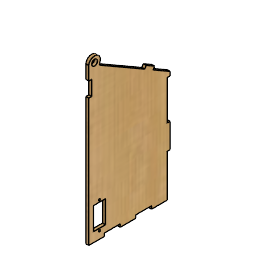
GREENHOUSE ASSEMBLY ALTERED (Autodesk Fusion 360 archive; units mm, degrees)
design "RIght"
Autodesk Fusion 360 part; units mm, degrees
(part 1 of 25)
sketch "Sketch1" plane through (150, 0, 0) normal (1, 0, 0) x (0, 1, 0)
  line L0 (64, 0) -> (80, 0)
  line L1 (80, 0) -> (80, 3)
  line L2 (80, 3) -> (64, 3) construction
  line L3 (0, 3) -> (0, 0)
  line L4 (0, 3) -> (0, 160)
  line L5 (0, 160) -> (83, 112.0799)
  line L6 (80, 3) -> (80, 108.0799)
  line L7 (80, 108.0799) -> (83, 108.0799)
  line L8 (83, 108.0799) -> (83, 112.0799)
  circle A0 centre (5.9574, 158.3503) radius 2.9841
  line L9 (4.524, 160.9676) -> (8.9408, 158.4176) construction
  line L10 (8.9408, 158.4176) -> (7.3908, 155.7329) construction
  line L11 (7.3908, 155.7329) -> (2.974, 158.2829) construction
  line L12 (2.974, 158.2829) -> (4.524, 160.9676) construction
  arc A1 (11.1398, 155.3582) -> (0, 157.7854) centre (5.9574, 158.3503) ccw
  line L13 (-5.009, 151.3242) -> (0, 160) construction
  line L14 (11.1398, 155.3582) -> (10.3648, 154.0159) construction
  arc A2 (11.1398, 155.3582) -> (11.7071, 153.2409) centre (12.4821, 154.5832) ccw
  line L15 (64, 3) -> (64, 0)
  line L16 (0, 0) -> (16, 0)
  line L17 (16, 0) -> (16, 3)
  line L18 (80, 0) -> (80, 3)
  line L19 (64, 0) -> (80, 0)
  line L20 (64, 0) -> (64, 3)
  line L21 (48, 3) -> (64, 3)
  line L22 (48, 0) -> (48, 3)
  line L23 (32, 0) -> (48, 0)
  line L24 (32, 0) -> (32, 3)
  line L25 (16, 3) -> (32, 3)
  line L26 (57.0192, 127.0799) -> (58.5192, 129.678)
  line L27 (58.5192, 129.678) -> (67.1795, 124.678)
  line L28 (67.1795, 124.678) -> (65.6795, 122.0799)
  line L29 (0, 145) -> (3, 145)
  line L30 (3, 145) -> (3, 130)
  line L31 (3, 130) -> (0, 130)
  line L32 (80, 68.04) -> (83, 68.04)
  line L33 (83, 68.04) -> (83, 43.04)
  line L34 (83, 43.04) -> (80, 43.04)
  line L35 (83, 55.54) -> (80, 55.54) construction
  dimension "d13" = 60
  dimension "d14" = 160
  dimension "d22" = 3
  dimension "d23" = 4
  dimension "d24" = 3.1
  dimension "d25" = 5.1
  dimension "d26" = 3
  dimension "d45" = 3
  dimension "d46" = 10
  dimension "d47" = 20
  dimension "d54" = 3
  dimension "d55" = 15
  dimension "d56" = 15
  dimension "d60" = 25
  constraint perpendicular L2 L4
  constraint coincident L1.end L2.start
  constraint perpendicular L2 L6
  constraint perpendicular L6 L7
  constraint perpendicular L7 L8
  constraint perpendicular L9 L10
  constraint parallel L9 L11
  constraint parallel L10 L12
  constraint coincident A0 L9.end
  constraint coincident A0 L9.start
  constraint coincident A0 L10.end
  constraint collinear L5 L11
  constraint coincident A0.centre A1.centre
  constraint coincident L5 L14.end
  constraint tangent A1 L14
  constraint perpendicular L5 L13
  constraint perpendicular L5 L14
  constraint tangent A1 L13
  constraint coincident L4 A1.end
  constraint tangent A1 A2
  constraint tangent L5 A2
  constraint coincident L5 A2.end
  constraint coincident L3.start L4.start
  constraint coincident L5 L26.start
  constraint perpendicular L5 L26
  constraint perpendicular L26 L27
  constraint coincident L5 L28.end
  constraint perpendicular L5 L28
  constraint coincident L4 L29.start
  constraint perpendicular L4 L29
  constraint perpendicular L29 L30
  constraint coincident L4 L31.end
  constraint perpendicular L4 L31
  constraint coincident L6 L32.start
  constraint perpendicular L6 L32
  constraint perpendicular L32 L33
  constraint coincident L6 L34.end
  constraint perpendicular L6 L34
  constraint collinear L8 L33
  constraint midpoint L33 L35.start
  constraint midpoint L6 L35.end
  constraint perpendicular L33 L35
  measures "d13" angle of L4 L5
  measures "d14" distance of L3.end L4.end
  measures "d22" distance of L6.end L7.end
  measures "d23" distance of L5.end L7.end
  measures "d24" distance of L9.end L10.end
  measures "d25" distance of L9.start L9.end
  measures "d26" distance of A0 A1
  measures "d45" distance of L26.start L26.end
  measures "d46" distance of L26.end L27.end
  measures "d47" distance of L5.end L28
  measures "d54" distance of L29.start L29.end
  measures "d55" distance of L29.end L30.end
  measures "d56" distance of L4.end L29
  measures "d60" distance of L32.end L33.end
extrude "Extrude1" add sketch "Sketch1" along normal blind 3 contours L0 L1 L3 L4 L5 L6 L7 L8 A0 A1 L15 L16 L17 L18 L19 L20 L21 L22 L23 L24 L25 L29 L30 L31 | L6 L32 L33 L34 | L5 L26 L27 L28 | L5 A0 A1 A2
sketch "Sketch2" plane through (153, 0, 0) normal (1, 0, 0) x (0, 1, 0)
  circle A0 centre (5.9574, 158.3503) radius 2.9841
  line L0 (80, 68.04) -> (80, 108.0799)
  line L1 (80, 108.0799) -> (83, 108.0799)
  line L2 (83, 108.0799) -> (83, 112.0799)
  line L3 (83, 112.0799) -> (65.6795, 122.0799)
  line L4 (65.6795, 122.0799) -> (67.1795, 124.678)
  line L5 (67.1795, 124.678) -> (58.5192, 129.678)
  line L6 (58.5192, 129.678) -> (57.0192, 127.0799)
  line L7 (57.0192, 127.0799) -> (11.7071, 153.2409)
  arc A1 (11.1398, 155.3582) -> (11.7071, 153.2409) centre (12.4821, 154.5832) ccw
  arc A2 (11.1398, 155.3582) -> (0, 158.9152) centre (5.9574, 158.3503) ccw
  line L8 (0, 158.9152) -> (0, 145)
  line L9 (0, 145) -> (3, 145)
  line L10 (3, 145) -> (3, 130)
  line L11 (3, 130) -> (0, 130)
  line L12 (0, 130) -> (0, 0)
  line L13 (0, 0) -> (16, 0)
  line L14 (16, 0) -> (16, 3)
  line L15 (16, 3) -> (32, 3)
  line L16 (32, 3) -> (32, 0)
  line L17 (32, 0) -> (48, 0)
  line L18 (48, 0) -> (48, 3)
  line L19 (48, 3) -> (64, 3)
  line L20 (64, 3) -> (64, 0)
  line L21 (64, 0) -> (80, 0)
  line L22 (80, 0) -> (80, 43.04)
  line L23 (80, 43.04) -> (83, 43.04)
  line L24 (83, 43.04) -> (83, 68.04)
  line L25 (83, 68.04) -> (80, 68.04)
  arc A3 (10.3278, 35.6711) -> (11.6278, 35.6711) centre (10.9778, 34.9111) ccw
  arc A4 (11.6278, 6.8512) -> (10.3278, 6.8512) centre (10.9778, 7.6111) ccw
  arc A5 (10.3278, 6.8512) -> (11.6278, 6.8512) centre (10.9778, 7.6111) ccw
  arc A6 (11.6278, 35.6711) -> (10.3278, 35.6711) centre (10.9778, 34.9111) ccw
  line L26 (16.8528, 26.6361) -> (16.8528, 10.0111) construction
  line L27 (16.8528, 32.5111) -> (16.8528, 26.6361) construction
  line L28 (10.9778, 32.5111) -> (16.8528, 32.5111) construction
  line L29 (5.1028, 32.5111) -> (10.9778, 32.5111) construction
  line L30 (5.1028, 26.6361) -> (5.1028, 32.5111) construction
  line L31 (5.1028, 10.0111) -> (5.1028, 26.6361) construction
  line L32 (5.1028, 10.0111) -> (16.8528, 10.0111) construction
  line L33 (4.9028, 9.8111) -> (17.0528, 9.8111)
  line L34 (17.0528, 26.6361) -> (17.0528, 9.8111)
  line L35 (17.0528, 32.7111) -> (17.0528, 26.6361)
  line L36 (10.9778, 32.7111) -> (17.0528, 32.7111)
  line L37 (4.9028, 32.7111) -> (10.9778, 32.7111)
  line L38 (4.9028, 26.6361) -> (4.9028, 32.7111)
  line L39 (4.9028, 9.8111) -> (4.9028, 26.6361)
  dimension "d94" = 0.2
  constraint coincident A4.start A5.end
  constraint coincident A4.centre A5.centre
  constraint coincident A3.end A6.start
  constraint coincident A3.centre A6.centre
  constraint coincident A3.start A6.end
  constraint coincident A4.end A5.start
extrude "Extrude2" cut sketch "Sketch2" against normal up to surface (3 mm away) contours A3 A6 | A4 A5 | L33 L34 L35 L36 L37 L38 L39

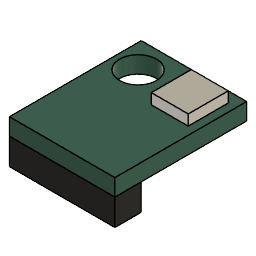
design "BMP180"
Autodesk Fusion 360 part; units mm, degrees
sketch "Sketch1" plane through (0, 0, 0) normal (0, 0, 1) x (1, 0, 0)
  line L0 (0, 0) -> (10, 0)
  line L1 (10, 0) -> (10, 12.5)
  line L2 (10, 12.5) -> (0, 12.5)
  line L3 (0, 12.5) -> (0, 0)
  circle A0 centre (2.25, 9.95) radius 1.75
  line L4 (5.75, 11.5) -> (9.25, 11.5)
  line L5 (9.25, 11.5) -> (9.25, 7.7)
  line L6 (9.25, 7.7) -> (5.75, 7.7)
  line L7 (5.75, 7.7) -> (5.75, 11.5)
  line L8 (10, 2.5) -> (0, 2.5)
  dimension "d1" = 10
  dimension "d2" = 12.5
  dimension "d3" = 3.5
  dimension "d4" = 2.55
  dimension "d5" = 2.25
  dimension "d6" = 3.5
  dimension "d7" = 3.8
  dimension "d8" = 0.75
  dimension "d9" = 1
  dimension "d10" = 2.5
  constraint horizontal L0
  constraint vertical L1
  constraint horizontal L2
  constraint vertical L3
  constraint coincident L0.start L3.end
  constraint horizontal L4
  constraint vertical L5
  constraint horizontal L6
  constraint vertical L7
  constraint coincident L1 L8.start
  constraint coincident L3 L8.end
  constraint perpendicular L3 L8
  measures "d1" distance of L0.start L0.end
  measures "d2" distance of L0.start L2.end
  measures "d3" diameter of A0
  measures "d4" distance of L2 A0.centre
  measures "d5" distance of L3 A0.centre
  measures "d6" distance of L4.start L4.end
  measures "d7" distance of L4.start L6.end
  measures "d8" distance of L1 L5
  measures "d9" distance of L2 L4
  measures "d10" distance of L0 L8
extrude "Extrude1" add sketch "Sketch1" along normal blind 1.6 contours L0 L1 L3 L8 | L1 L2 L3 L8 | L4 L5 L6 L7 makes body 1
extrude "Extrude2" add sketch "Sketch1" along normal blind 1 from surface at 1.6 separate body contours L4 L5 L6 L7 makes body 2
extrude "Extrude3" add sketch "Sketch1" against normal blind 2.5 separate body contours L0 L1 L3 L8 makes body 3
equation "d4 = d3 / 2 + 0.8 mm"
equation "d5 = d3 / 2 + 0.5 mm"

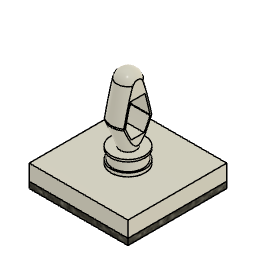
design "PCB Support Pin"
Autodesk Fusion 360 part; units mm, degrees
sketch "Sketch1" plane through (0, 0, 0) normal (0, 0, 1) x (1, 0, 0)
  line L0 (6.35, 6.35) -> (-6.35, 6.35)
  line L1 (-6.35, 6.35) -> (-6.35, -6.35)
  line L2 (-6.35, -6.35) -> (6.35, -6.35)
  line L3 (6.35, -6.35) -> (6.35, 6.35)
  line L4 (6.35, 6.35) -> (-6.35, -6.35) construction
  line L5 (-6.35, 6.35) -> (6.35, -6.35) construction
  dimension "d1" = 12.7
  dimension "d2" = 12.7
  constraint horizontal L0
  constraint perpendicular L0 L1
  constraint parallel L0 L2
  constraint parallel L1 L3
  constraint coincident L4 origin
  constraint coincident L5 origin
  measures "d1" distance of L1.end L2.end
  measures "d2" distance of L0.end L1.end
extrude "Extrude1" add sketch "Sketch1" along normal blind 2.032 makes body 1
extrude "Extrude2" add 1 faces at (-2.1167, -2.1167, 0) along direction (0, 0, -1) blind 0.8 separate body on bodies 1 makes body 2
sketch "Sketch2" plane through (0, 0, 0) normal (0, 1, 0) x (1, 0, 0)
  line L0 (-6.35, -2.032) -> (6.35, -2.032)
  line L1 (0, -2.032) -> (0, -12.6938)
  line L2 (0, -3.9625) -> (2.1828, -3.9625)
  line L3 (2.1828, -3.9625) -> (2.1828, -3.6971)
  line L4 (2.1828, -3.6971) -> (1.9857, -3.6971)
  line L5 (1.9857, -3.6971) -> (1.9857, -2.4654)
  line L6 (1.9857, -2.4654) -> (2.1828, -2.4654)
  line L7 (2.1828, -2.4654) -> (2.1828, -2.032)
  line L8 (6.35, 0.8) -> (-6.35, 0.8) construction
  line L9 (1.0176, -3.9625) -> (2.1587, -7.0975)
  line L10 (2.1763, -7.3064) -> (1.4028, -11.5248)
  arc A0 (0, -12.6938) -> (1.4028, -11.5248) centre (0, -11.2676) ccw
  arc A1 (2.1763, -7.3064) -> (2.1587, -7.0975) centre (1.7828, -7.2343) ccw
  line L11 (0, -12.6938) -> (1.1885, -12.6938) construction
  line L12 (1.1885, -12.6938) -> (1.4028, -11.5248) construction
  line L13 (2.1828, -3.9625) -> (2.1828, -7.2343) construction
  line L14 (1.6, -3.9625) -> (1.6, -5.5625) construction
  line L15 (1.6, -5.5625) -> (0, -5.5625) construction
  arc A2 (1.9795, -7.2704) -> (1.9708, -7.1659) centre (1.7828, -7.2343) ccw
  line L16 (0.8297, -4.0309) -> (0.8048, -3.9625)
  dimension "d7" = 4.7625
  dimension "d8" = 4.3656
  dimension "d10" = 0.4
  dimension "d11" = 8.7313
  dimension "d12" = 3.2
  dimension "d13" = 1.6
  dimension "d15" = 70
  constraint midpoint L0 L1.start
  constraint perpendicular L0 L1
  constraint perpendicular L1 L2
  constraint perpendicular L2 L3
  constraint perpendicular L3 L4
  constraint perpendicular L4 L5
  constraint perpendicular L5 L6
  constraint coincident L0 L7.end
  constraint perpendicular L0 L7
  constraint collinear L3 L7
  constraint coincident L2.start L1
  constraint coincident L1.end A0.start
  constraint tangent L10 A0
  constraint tangent L9 A1
  constraint tangent L10 A1
  constraint perpendicular L1 L11
  constraint tangent A0 L12
  constraint tangent A0 L11
  constraint coincident A1 L13.end
  constraint tangent A1 L13
  constraint perpendicular L2 L13
  constraint coincident L2 L9.start
  constraint coincident L2 L14.start
  constraint coincident L9 L14.end
  constraint perpendicular L2 L14
  constraint coincident L1 L15.end
  constraint perpendicular L1 L15
  constraint coincident L2 L16.end
  constraint concentric A1 A2
  measures "d7" distance of L2 L8
  measures "d10" radius of A1
  measures "d11" distance of L2 L1.end
  measures "d13" distance of L14.start L14.end
  measures "d15" angle of L2 L9
revolve "Revolve1" add sketch "Sketch2" angle 360 about axis through (0, 0, 2.032) along (0, 0, 1) bodies 1
sketch "Sketch3" plane through (0, 0, 0) normal (0, 1, 0) x (1, 0, 0)
  line L0 (-2.1828, -3.9625) -> (2.1828, -3.9625)
  arc A0 (-1.4028, -11.5248) -> (0, -12.6938) centre (0, -11.2676) ccw
  arc A1 (0, -12.6938) -> (1.4028, -11.5248) centre (0, -11.2676) ccw
  line L1 (1.25, -3.9625) -> (1.25, -12.6938)
  line L2 (1.25, -12.6938) -> (-1.25, -12.6938)
  line L3 (-1.25, -12.6938) -> (-1.25, -3.9625)
  line L4 (2.1828, -3.9625) -> (2.1828, -12.6938)
  line L5 (2.1828, -12.6938) -> (1.25, -12.6938)
  line L6 (-1.25, -12.6938) -> (-2.1828, -12.6938)
  line L7 (-2.1828, -12.6938) -> (-2.1828, -3.9625)
  dimension "d16" = 2.5
  constraint coincident L0 L1.start
  constraint perpendicular L0 L1
  constraint perpendicular L1 L2
  constraint coincident L0 L3.end
  constraint perpendicular L0 L3
  constraint midpoint A0.end L2
  constraint coincident L0.end L4.start
  constraint perpendicular L0 L4
  constraint perpendicular L1 L5
  constraint perpendicular L3 L6
  constraint coincident L0.start L7.end
  constraint perpendicular L0 L7
  measures "d16" distance of L1.end L2.end
extrude "Extrude3" cut sketch "Sketch3" along normal through all and the other way through all contours L0 L3 L6 L7 | L0 L1 L4 L5 bodies 1
sketch "Sketch4" plane through (1.25, 0, 0) normal (1, 0, 0) x (0, 1, 0)
  arc A0 (0.6367, 11.5248) -> (-0.6367, 11.5248) centre (0, 11.2676) ccw
  spline S0 degree 2 poles (-1.7815, 7.3064) (-1.0854, 10.4141) (-0.6367, 11.5248) knots 0 0 0 0.437351 0.437351 0.437351 weights 1 1.055449 1
  spline S1 degree 3 poles (-1.76, 7.0975) (-1.7782, 7.1383) (-1.7895, 7.19) (-1.7895, 7.2343) (-1.7895, 7.2572) (-1.7869, 7.2821) (-1.7815, 7.3064) knots -0.013287 -0.013287 -0.013287 -0.013287 0 0 0 0.006866 0.006866 0.006866 0.006866
  spline S2 degree 2 poles (0, 4.6009) (-0.6454, 4.6009) (-1.76, 7.0975) knots 0.311685 0.311685 0.311685 0.623369 0.623369 0.623369 weights 1 1.16768 1
  spline S3 degree 2 poles (1.76, 7.0975) (0.6454, 4.6009) (0, 4.6009) knots 0 0 0 0.311685 0.311685 0.311685 weights 1 1.16768 1
  spline S4 degree 3 poles (1.7815, 7.3064) (1.7869, 7.2821) (1.7895, 7.2572) (1.7895, 7.2343) (1.7895, 7.19) (1.7782, 7.1383) (1.76, 7.0975) knots -0.006866 -0.006866 -0.006866 -0.006866 0 0 0 0.013287 0.013287 0.013287 0.013287
  spline S5 degree 2 poles (0.6367, 11.5248) (1.0854, 10.4141) (1.7815, 7.3064) knots 0 0 0 0.437351 0.437351 0.437351 weights 1 1.055449 1
  spline S6 degree 3 poles (1.5773, 7.179) (1.0909, 6.0894) (0.7682, 5.5108) (0.4944, 5.1632) (0.2828, 4.8944) (0.1228, 4.8009) (0, 4.8009) knots 0 0 0 0 0.17577 0.17577 0.17577 0.311685 0.311685 0.311685 0.311685
  spline S7 degree 3 poles (0, 4.8009) (-0.1696, 4.8009) (-0.4174, 4.9925) (-0.7546, 5.5437) (-0.9772, 5.9076) (-1.2343, 6.4106) (-1.5773, 7.179) knots 0.311685 0.311685 0.311685 0.311685 0.499423 0.499423 0.499423 0.623369 0.623369 0.623369 0.623369
  spline S8 degree 3 poles (-1.5773, 7.179) (-1.5825, 7.1906) (-1.5895, 7.2239) (-1.5895, 7.2343) (-1.5895, 7.2423) (-1.5883, 7.2538) (-1.5863, 7.2627) knots -0.013287 -0.013287 -0.013287 -0.013287 0 0 0 0.006866 0.006866 0.006866 0.006866
  spline S9 degree 3 poles (-1.5863, 7.2627) (-1.1749, 9.0993) (-0.8714, 10.2577) (-0.6005, 11.0468) (-0.5494, 11.1956) (-0.4997, 11.3299) (-0.4512, 11.4499) knots 0 0 0 0 0.367958 0.367958 0.367958 0.437351 0.437351 0.437351 0.437351
  arc A1 (0.4512, 11.4499) -> (-0.4512, 11.4499) centre (0, 11.2676) ccw
  spline S10 degree 3 poles (0.4512, 11.4499) (0.7082, 10.8137) (0.9931, 9.8115) (1.3651, 8.2283) (1.4352, 7.9297) (1.5087, 7.6091) (1.5863, 7.2627) knots 0 0 0 0 0.367958 0.367958 0.367958 0.437351 0.437351 0.437351 0.437351
  spline S11 degree 3 poles (1.5863, 7.2627) (1.5883, 7.2538) (1.5895, 7.2423) (1.5895, 7.2343) (1.5895, 7.2239) (1.5825, 7.1906) (1.5773, 7.179) knots -0.006866 -0.006866 -0.006866 -0.006866 0 0 0 0.013287 0.013287 0.013287 0.013287
  line L0 (0.8161, 5.6442) -> (-0.8149, 5.6442)
  line L1 (0.9353, 9.9416) -> (-0.9355, 9.9416)
  dimension "d18" = 0.2
  constraint coincident S6 L0.start
  constraint coincident S7 L0.end
  constraint horizontal L0
  constraint coincident S10 L1.start
  constraint coincident S9 L1.end
  constraint parallel L0 L1
extrude "Extrude4" cut sketch "Sketch4" against normal through all contours S6 S7 S8 S9 S10 S11 L0 L1 bodies 1
equation "d7 = 3\" / 16"
equation "d8 = 11\" / 64"
equation "d11 = 11\" / 32"

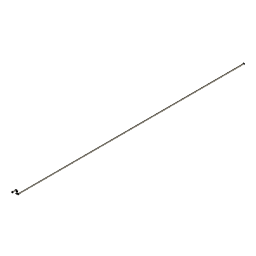
design "Push Rod"
Autodesk Fusion 360 part; units mm, degrees
sketch "Sketch1" plane through (0, 0, 0) normal (1, 0, 0) x (0, 1, 0)
  line L0 (0, 0) -> (3, 0)
  line L1 (4, -1) -> (4, -3)
  line L2 (5, -4) -> (204, -4)
  arc A0 (4, -1) -> (3, 0) centre (3, -1) ccw
  arc A1 (4, -3) -> (5, -4) centre (5, -3) ccw
  point P0 (4, 0)
  point P1 (4, -4)
  dimension "d1" = 4
  dimension "d2" = 4
  dimension "d3" = 200
  dimension "d4" = 1
  dimension "d5" = 1
  constraint coincident L0.start origin
  constraint horizontal L0
  constraint perpendicular L0 L1
  constraint perpendicular L1 L2
  constraint coincident P0 L0
  constraint coincident P0 L1
  constraint tangent L0 A0
  constraint tangent L1 A0
  constraint coincident P1 L1
  constraint coincident P1 L2
  constraint tangent L1 A1
  constraint tangent L2 A1
  measures "d1" distance of L0.start P0
  measures "d2" distance of P0 P1
  measures "d3" distance of P1 L2.end
  measures "d4" radius of A0
  measures "d5" radius of A1
sketch "Sketch2" plane through (0, 0, 0) normal (0, 1, 0) x (1, 0, 0)
  circle A0 centre (0, 0) radius 0.6
  dimension "d6" = 1.2
  constraint coincident A0.centre origin
  measures "d6" diameter of A0
sweep "Sweep1" add profiles "Sketch2" path "Sketch1" along L0 A0 L1 A1 L2 section 1

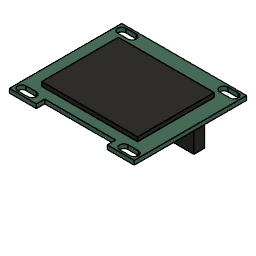
design "oled"
description: IIC OLED 0.96" 4Pin SSD1306
part number: GME12864-11
Autodesk Fusion 360 part; units mm, degrees
sketch "Sketch1" plane through (0, 0, 0) normal (0, 1, 0) x (1, 0, 0)
  line L0 (0, 0) -> (30, 0)
  line L1 (30, 0) -> (30, -27)
  line L2 (30, -27) -> (0, -27)
  line L3 (0, -27) -> (0, 0)
  line L4 (6.5, -27) -> (6.5, -25)
  line L5 (6.5, -25) -> (23.5, -25)
  line L6 (23.5, -25) -> (23.5, -27)
  line L7 (15, -27) -> (15, -25) construction
  line L8 (3.5, -4.3) -> (26.5, -4.3)
  line L9 (26.5, -4.3) -> (26.5, -22.7)
  line L10 (26.5, -22.7) -> (3.5, -22.7)
  line L11 (3.5, -22.7) -> (3.5, -4.3)
  line L12 (1.5, -2.5) -> (4, -2.5)
  arc A0 (4, -2.5) -> (4, -0.5) centre (4, -1.5) ccw
  line L13 (4, -0.5) -> (1.5, -0.5)
  arc A1 (1.5, -0.5) -> (1.5, -2.5) centre (1.5, -1.5) ccw
  line L14 (1.5, -1.5) -> (4, -1.5) construction
  line L15 (15, 0) -> (15, -25) construction
  line L16 (0, -13.5) -> (30, -13.5) construction
  arc A2 (26, -0.5) -> (26, -2.5) centre (26, -1.5) ccw
  line L17 (26, -0.5) -> (28.5, -0.5)
  arc A3 (28.5, -2.5) -> (28.5, -0.5) centre (28.5, -1.5) ccw
  line L18 (28.5, -2.5) -> (26, -2.5)
  line L19 (26, -26.5) -> (28.5, -26.5)
  arc A4 (28.5, -26.5) -> (28.5, -24.5) centre (28.5, -25.5) ccw
  line L20 (28.5, -24.5) -> (26, -24.5)
  arc A5 (26, -24.5) -> (26, -26.5) centre (26, -25.5) ccw
  line L21 (4, -26.5) -> (1.5, -26.5)
  arc A6 (4, -26.5) -> (4, -24.5) centre (4, -25.5) ccw
  arc A7 (1.5, -24.5) -> (1.5, -26.5) centre (1.5, -25.5) ccw
  line L22 (1.5, -24.5) -> (4, -24.5)
  dimension "d1" = 30
  dimension "d2" = 27
  dimension "d3" = 6.5
  dimension "d4" = 2
  dimension "d5" = 3.5
  dimension "d6" = 3.5
  dimension "d7" = 4.3
  dimension "d8" = 4.3
  dimension "d22" = 1.5
  dimension "d23" = 1.5
  dimension "d24" = 1
  dimension "d25" = 2.5
  constraint horizontal L0
  constraint vertical L1
  constraint horizontal L2
  constraint vertical L3
  constraint coincident L0.start L3.end
  constraint coincident L2 L4.start
  constraint perpendicular L2 L4
  constraint perpendicular L4 L5
  constraint coincident L2 L6.end
  constraint perpendicular L2 L6
  constraint midpoint L2 L7.start
  constraint midpoint L5 L7.end
  constraint perpendicular L2 L7
  constraint horizontal L8
  constraint vertical L9
  constraint horizontal L10
  constraint vertical L11
  constraint tangent L12 A0
  constraint tangent A0 L13
  constraint parallel L12 L13
  constraint tangent L13 A1
  constraint tangent L12 A1
  constraint horizontal L14
  constraint midpoint L0 L15.start
  constraint midpoint L3 L16.start
  constraint midpoint L1 L16.end
  constraint symmetric L12.start L15 A3.start
  constraint symmetric L12.end L15 A2.end
  constraint symmetric A0.end L15 A2.start
  constraint symmetric L13.end L15 L17.end
  constraint symmetric A0 L15 A2
  constraint symmetric A1 L15 A3
  constraint symmetric L12.start L16 A7.start
  constraint symmetric L12.end L16 A6.end
  constraint symmetric A0.end L16 L21.start
  constraint symmetric L13.end L16 L21.end
  constraint symmetric A0 L16 A6
  constraint symmetric A1 L16 A7
  constraint symmetric L16 A2.end L20.end
  constraint symmetric L16 A2.start L19.start
  constraint symmetric L16 A2 A5
  constraint symmetric L16 L17.end L19.end
  constraint symmetric L16 A3.start A4.end
  constraint symmetric L16 A3 A4
  measures "d1" distance of L0.start L0.end
  measures "d2" distance of L0.start L2.end
  measures "d3" distance of L1 L6
  measures "d4" distance of L2 L5
  measures "d5" distance of L1 L9
  measures "d6" distance of L3 L11
  measures "d7" distance of L0 L8
  measures "d8" distance of L2 L10
  measures "d22" distance of L3 A1.centre
  measures "d23" distance of L0 A1.centre
  measures "d24" radius of A1
  measures "d25" distance of A1.centre A0.centre
extrude "Extrude1" add sketch "Sketch1" along normal blind 1 contours L8 L9 L10 L11 makes body 1
extrude "Extrude2" add sketch "Sketch1" against normal blind 1 separate body contours L0 L1 L2 L3 L4 L5 L6 | L8 L9 L10 L11 makes body 2
sketch "Sketch2" plane through (0, -1, 0) normal (0, -1, 0) x (1, 0, 0)
  line L0 (6.5, 25) -> (6.5, 27)
  line L1 (6.5, 27) -> (0, 27)
  line L2 (0, 27) -> (0, 0)
  line L3 (0, 0) -> (30, 0)
  line L4 (30, 0) -> (30, 27)
  line L5 (30, 27) -> (23.5, 27)
  line L6 (23.5, 27) -> (23.5, 25)
  line L7 (23.5, 25) -> (6.5, 25)
  line L8 (10.1, 2.6) -> (19.9, 2.6)
  line L9 (19.9, 2.6) -> (19.9, 0)
  line L10 (10.1, 0) -> (10.1, 2.6)
  line L11 (15, 0) -> (15, 2.6) construction
  arc A0 (26, 2.5) -> (26, 0.5) centre (26, 1.5) ccw
  line L12 (26, 2.5) -> (28.5, 2.5)
  arc A1 (28.5, 0.5) -> (28.5, 2.5) centre (28.5, 1.5) ccw
  line L13 (28.5, 0.5) -> (26, 0.5)
  arc A2 (26, 26.5) -> (26, 24.5) centre (26, 25.5) ccw
  line L14 (26, 26.5) -> (28.5, 26.5)
  arc A3 (28.5, 24.5) -> (28.5, 26.5) centre (28.5, 25.5) ccw
  line L15 (28.5, 24.5) -> (26, 24.5)
  arc A4 (4, 24.5) -> (4, 26.5) centre (4, 25.5) ccw
  line L16 (4, 24.5) -> (1.5, 24.5)
  arc A5 (1.5, 26.5) -> (1.5, 24.5) centre (1.5, 25.5) ccw
  line L17 (1.5, 26.5) -> (4, 26.5)
  arc A6 (1.5, 2.5) -> (1.5, 0.5) centre (1.5, 1.5) ccw
  line L18 (1.5, 2.5) -> (4, 2.5)
  arc A7 (4, 0.5) -> (4, 2.5) centre (4, 1.5) ccw
  line L19 (4, 0.5) -> (1.5, 0.5)
  dimension "d13" = 9.8
  dimension "d14" = 2.6
  constraint horizontal L8
  constraint vertical L9
  constraint vertical L10
  constraint midpoint L3 L11.start
  constraint perpendicular L3 L11
  constraint coincident L3 L9.end
  constraint coincident L3 L10.start
  constraint midpoint L8 L11.end
  measures "d13" distance of L8.start L8.end
  measures "d14" distance of L8.start L10.start
extrude "Extrude3" add sketch "Sketch2" along normal blind 15 separate body contours L3 L8 L9 L10 makes body 3
sketch "Minimal Projection" plane through (0, -1, 0) normal (0, -1, 0) x (1, 0, 0)
  arc A0 (26, 2.5) -> (26, 0.5) centre (26, 1.5) ccw
  line L0 (26, 2.5) -> (28.5, 2.5)
  arc A1 (28.5, 0.5) -> (28.5, 2.5) centre (28.5, 1.5) ccw
  line L1 (28.5, 0.5) -> (26, 0.5)
  arc A2 (26, 26.5) -> (26, 24.5) centre (26, 25.5) ccw
  line L2 (26, 26.5) -> (28.5, 26.5)
  arc A3 (28.5, 24.5) -> (28.5, 26.5) centre (28.5, 25.5) ccw
  line L3 (28.5, 24.5) -> (26, 24.5)
  arc A4 (4, 24.5) -> (4, 26.5) centre (4, 25.5) ccw
  line L4 (4, 24.5) -> (1.5, 24.5)
  arc A5 (1.5, 26.5) -> (1.5, 24.5) centre (1.5, 25.5) ccw
  line L5 (1.5, 26.5) -> (4, 26.5)
  arc A6 (1.5, 2.5) -> (1.5, 0.5) centre (1.5, 1.5) ccw
  line L6 (1.5, 2.5) -> (4, 2.5)
  arc A7 (4, 0.5) -> (4, 2.5) centre (4, 1.5) ccw
  line L7 (4, 0.5) -> (1.5, 0.5)
  line L8 (6.5, 25) -> (6.5, 27)
  line L9 (6.5, 27) -> (0, 27)
  line L10 (0, 27) -> (0, 0)
  line L11 (0, 0) -> (30, 0)
  line L12 (30, 0) -> (30, 27)
  line L13 (30, 27) -> (23.5, 27)
  line L14 (23.5, 27) -> (23.5, 25)
  line L15 (23.5, 25) -> (6.5, 25)
  line L16 (19.9, 0) -> (19.9, 2.6)
  line L17 (19.9, 2.6) -> (10.1, 2.6)
  line L18 (10.1, 2.6) -> (10.1, 0)

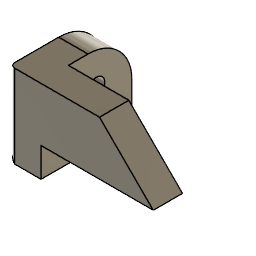
design "MOUNT REAl"
part number: 2026-05-05-22-33-46-720
Autodesk Fusion 360 part; units mm, degrees
sketch "Sketch1" plane through (0, 0, 0) normal (0, 0, 1) x (1, 0, 0)
  line L0 (0, 0) -> (14.68, 0)
  line L1 (14.68, 0) -> (14.68, 3)
  line L2 (14.68, 3) -> (11.68, 3)
  line L3 (11.68, 3) -> (3, 3)
  line L4 (3, 3) -> (3, 9.502)
  line L5 (0, 0) -> (0, 9.502)
  line L6 (0, 9.502) -> (3, 9.502)
  dimension "d4" = 3
  dimension "d5" = 3
  dimension "d6" = 8.68
  dimension "d7" = 6.502
  dimension "d88" = 3
  constraint coincident L0.start L5.start
  constraint horizontal L0
  constraint perpendicular L0 L1
  constraint perpendicular L1 L2
  constraint parallel L2 L3
  constraint perpendicular L3 L4
  constraint perpendicular L0 L5
  constraint perpendicular L4 L6
  measures "d4" distance of L0.end L1.end
  measures "d5" distance of L1.end L2.end
  measures "d6" distance of L2.end L3.end
  measures "d7" distance of L3.end L4.end
  measures "d88" distance of L4.end L5.end
extrude "Extrude18" add sketch "Sketch1" along normal blind 8.5 makes body 1
sketch "Sketch18" plane through (0, 0, 0) normal (0, -1, 0) x (1, 0, 0)
  line L0 (0, 0) -> (14.68, 0)
  line L1 (14.68, 0) -> (14.68, 8.5)
  line L2 (14.68, 8.5) -> (0, 8.5)
  line L3 (0, 8.5) -> (0, 0)
  line L4 (3.2, 0) -> (10.41, 0)
  line L5 (10.41, 0) -> (10.41, 3)
  line L6 (10.41, 3) -> (3.2, 3)
  line L7 (3.2, 3) -> (3.2, 0)
  dimension "d93" = 7.21
  dimension "d94" = 3
  dimension "d95" = 10.41
  constraint perpendicular L4 L5
  constraint perpendicular L5 L6
  constraint perpendicular L4 L7
  constraint coincident L0 L4.start
  constraint coincident L0 L4.end
  measures "d93" distance of L5.end L6.end
  measures "d94" distance of L4.end L5.end
  measures "d95" distance of L3 L5
extrude "Extrude19" cut sketch "Sketch18" against normal blind 3 contours L0 L4 L5 L6 L7 bodies 1
sketch "Sketch19" plane through (0, 0, 0) normal (0, 0, 1) x (1, 0, 0)
  line L0 (1.73, 2) -> (1.73, 8.5)
  line L1 (1.73, 8.5) -> (7.43, 8.5)
  line L2 (7.43, 8.5) -> (7.43, 2)
  line L3 (7.43, 2) -> (1.73, 2)
  dimension "d99" = 5.7
  constraint perpendicular L0 L1
  constraint perpendicular L1 L2
  measures "d99" distance of L0.end L1.end
sketch "Sketch23" plane through (0, 0, 0) normal (-1, 0, 0) x (0, -1, 0)
  line L0 (-9.502, 0) -> (0, 0)
  line L1 (0, 0) -> (0, 8.5)
  line L2 (0, 8.5) -> (-9.502, 8.5)
  line L3 (-9.502, 8.5) -> (-9.502, 0)
  circle A0 centre (-5.852, 5.15) radius 0.8695
  dimension "d107" = 1.739
  dimension "d108" = 3.35
  dimension "d109" = 3.65
  measures "d107" diameter of A0
  measures "d108" distance of L2 A0.centre
  measures "d109" distance of L3 A0.centre
extrude "Extrude23" cut sketch "Sketch23" against normal blind 6.5 contours A0 bodies 1
fillet "Fillet3" radius 4.5 1 edges at (1.5, 9.502, 8.5) on bodies 1
chamfer "Chamfer3" distance 0.5 angle 45 1 edges at (0, 4.751, 0) on bodies 1
fillet "Fillet4" radius 0.5 1 edges at (0, 0, 4.5) on bodies 1
chamfer "Chamfer4" distance 5.5 angle 45 1 edges at (14.68, 1.5, 8.5) on bodies 1
sketch "Sketch24" plane through (0, 0, 0) normal (0, 0, 1) x (1, 0, 0)
  line L0 (3, 3) -> (7, 3)
  line L1 (7, 3) -> (7, 9.5)
  line L2 (7, 9.5) -> (3, 9.5)
  line L3 (3, 9.5) -> (3, 3)
  dimension "d118" = 4
  dimension "d119" = 6.5
  dimension "d120" = 3
  dimension "d121" = 3
  constraint horizontal L0
  constraint perpendicular L0 L1
  constraint perpendicular L1 L2
  constraint perpendicular L0 L3
  measures "d118" distance of L0.start L0.end
  measures "d119" distance of L0 L2
  measures "d120" distance of origin L3
  measures "d121" distance of origin L0
extrude "Extrude24" add sketch "Sketch24" along normal blind 3 separate body makes body 2
sketch "Sketch25" plane through (7, 0, 0) normal (1, 0, 0) x (0, 1, 0)
  line L0 (3, 0) -> (9.5, 0)
  line L1 (9.5, 0) -> (9.5, 3)
  line L2 (9.5, 3) -> (3, 3)
  line L3 (3, 3) -> (3, 0)
  line L4 (3, 3) -> (9.5, 1.5)
  line L5 (9.5, 1.5) -> (3, 1.5)
  line L6 (3, 3) -> (3, 1.5)
  constraint coincident L2.end L3.start
  constraint midpoint L1 L4.end
  constraint midpoint L3 L5.end
extrude "Extrude25" cut sketch "Sketch25" against normal blind 2 contours L1 L2 L4 bodies 2
extrude "Extrude26" cut sketch "Sketch25" against normal blind 4 contours L1 L2 L4 bodies 2
sketch "Sketch26" plane through (0, 3, 0) normal (0, 1, 0) x (-1, 0, 0)
  line L0 (-9.18, 8.5) -> (-14.68, 3)
  line L1 (-14.68, 3) -> (-14.68, 0)
  line L2 (-14.68, 0) -> (-10.41, 0)
  line L3 (-10.41, 0) -> (-10.41, 3)
  line L4 (-10.41, 3) -> (-3.2, 3)
  line L5 (-3.2, 3) -> (-3.2, 0)
  line L6 (-3.2, 0) -> (-3, 0)
  line L7 (-3, 0) -> (-3, 8.5)
  line L8 (-3, 8.5) -> (-9.18, 8.5)
  line L9 (-10.41, 3) -> (-14.68, 3)
  line L10 (-14.68, 3) -> (-14.68, 0)
  line L11 (-10.41, 0) -> (-14.68, 0)
  line L12 (-10.41, 0) -> (-10.41, 3)
  constraint coincident L3.end L4.start
  constraint coincident L0.end L1.start
  constraint coincident L1.end L2.start
  constraint coincident L2.end L3.start
extrude "Extrude27" cut sketch "Sketch26" against normal blind 4 contours L1 L2 L3 L9 L10 L11 L12 bodies 1
extrude "Extrude28" cut 1 faces at (7, 5.1667, 1.5) along direction (-1, 0, 0) blind 3.8 on bodies 2 bodies 2

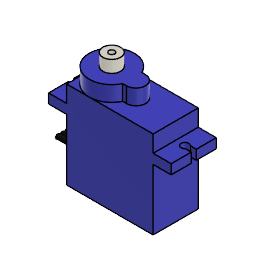
design "SG90 Micro Servo"
Autodesk Fusion 360 part; units mm, degrees
sketch "Sketch2" plane through (0, 0, 0) normal (0, 1, 0) x (1, 0, 0)
  line L0 (0, 0) -> (22.5, 0)
  line L1 (22.5, 0) -> (22.5, -22.75)
  line L2 (22.5, -22.75) -> (0, -22.75)
  line L3 (0, -22.75) -> (0, 0)
  line L4 (-4.7, -15.9) -> (-4.7, -18.4)
  line L5 (27.2, -18.4) -> (27.2, -15.9)
  line L6 (-4.7, -18.4) -> (0, -18.4)
  line L7 (22.5, -18.4) -> (27.2, -18.4)
  line L8 (27.2, -15.9) -> (22.5, -15.9)
  line L9 (0, -15.9) -> (-4.7, -15.9)
  dimension "d3" = 22.5
  dimension "d4" = 22.75
  dimension "d6" = 4.35
  dimension "d7" = 2.5
  dimension "d8" = 4.7
  dimension "d9" = 4.7
  constraint horizontal L0
  constraint vertical L1
  constraint horizontal L2
  constraint vertical L3
  constraint coincident L0.start L3.end
  constraint horizontal L8
  constraint vertical L4
  constraint horizontal L6
  constraint vertical L5
  constraint coincident L3 L6.end
  constraint coincident L1 L7.start
  constraint collinear L6 L7
  constraint coincident L1 L8.end
  constraint coincident L3 L9.start
  constraint collinear L8 L9
  measures "d3" distance of L0.start L0.end
  measures "d4" distance of L0.start L2.end
  measures "d6" distance of L2 L6
  measures "d7" distance of L5.end L5.start
  measures "d8" distance of L1 L5
  measures "d9" distance of L3 L4
extrude "Extrude2" add sketch "Sketch2" along normal blind 11.75 makes body 1
sketch "Sketch3" plane through (0, 0, 22.75) normal (0, 0, 1) x (-1, 0, 0)
  line L0 (0, 0) -> (-22.5, 0)
  line L1 (-22.5, 0) -> (-22.5, -11.75)
  line L2 (-22.5, -11.75) -> (0, -11.75)
  line L3 (0, -11.75) -> (0, 0)
  circle A0 centre (-5.875, -5.875) radius 5.875
  line L4 (-5.875, -5.875) -> (-12.175, -5.875) construction
  line L5 (-11.1915, -8.375) -> (-12.175, -8.375)
  line L6 (-11.1915, -3.375) -> (-12.175, -3.375)
  arc A1 (-12.175, -3.375) -> (-12.175, -8.375) centre (-12.175, -5.875) ccw
  dimension "d13" = 6.3
  dimension "d14" = 2.5
  constraint tangent L0 A0
  constraint tangent L2 A0
  constraint tangent L3 A0
  constraint coincident A0.centre L4.start
  constraint coincident L4.end A1.centre
  constraint horizontal L4
  constraint coincident A0 L5.start
  constraint tangent L5 A1
  constraint coincident A0 L6.start
  constraint tangent L6 A1
  constraint horizontal L5
  constraint horizontal L6
  measures "d13" distance of A0.centre L4.end
  measures "d14" radius of A1
extrude "Extrude3" add sketch "Sketch3" along normal blind 4 contours A0 | A0 L5 L6 A1 bodies 1
sketch "Sketch4" plane through (0, 0, 26.75) normal (0, 0, 1) x (-1, 0, 0)
  arc A0 (-11.1915, -8.375) -> (-11.1915, -3.375) centre (-5.875, -5.875) ccw
  line L0 (-11.1915, -3.375) -> (-12.175, -3.375)
  arc A1 (-12.175, -3.375) -> (-12.175, -8.375) centre (-12.175, -5.875) ccw
  line L1 (-12.175, -8.375) -> (-11.1915, -8.375)
  circle A2 centre (-5.875, -5.875) radius 2.3
  circle A3 centre (-5.875, -5.875) radius 0.75
  dimension "d17" = 4.6
  dimension "d28" = 1.5
  constraint concentric A0 A2
  constraint concentric A2 A3
  measures "d17" diameter of A2
  measures "d28" diameter of A3
extrude "Extrude4" add sketch "Sketch4" along normal blind 3.15 separate body contours A2 makes body 2
sketch "Sketch5" plane through (0, 0, 18.4) normal (0, 0, 1) x (-1, 0, 0)
  line L0 (4.7, 0) -> (0, 0)
  line L1 (0, 0) -> (0, -11.75)
  line L2 (0, -11.75) -> (4.7, -11.75)
  line L3 (4.7, -11.75) -> (4.7, 0)
  line L4 (-22.5, 0) -> (-27.2, 0)
  line L5 (-27.2, 0) -> (-27.2, -11.75)
  line L6 (-27.2, -11.75) -> (-22.5, -11.75)
  line L7 (-22.5, -11.75) -> (-22.5, 0)
  line L8 (-27.2, -5.875) -> (4.7, -5.875) construction
  line L9 (-11.25, -5.875) -> (-11.25, -0.3179)
  line L10 (4.7, -6.525) -> (3.1599, -6.525)
  line L11 (4.7, -5.225) -> (3.1599, -5.225)
  arc A0 (3.1599, -5.225) -> (3.1599, -6.525) centre (2.4, -5.875) ccw
  arc A1 (-25.6599, -6.525) -> (-25.6599, -5.225) centre (-24.9, -5.875) ccw
  line L12 (-27.2, -5.225) -> (-25.6599, -5.225)
  line L13 (-27.2, -6.525) -> (-25.6599, -6.525)
  dimension "d20" = 2
  dimension "d21" = 1.3
  dimension "d22" = 2.3
  constraint midpoint L5 L8.start
  constraint midpoint L3 L8.end
  constraint midpoint L8 L9.start
  constraint perpendicular L8 L9
  constraint coincident L8 A0.centre
  constraint coincident L3 L10.start
  constraint perpendicular L3 L10
  constraint coincident L3 L11.start
  constraint perpendicular L3 L11
  constraint symmetric L8 L10 L11
  constraint symmetric L9 L10.start L13.start
  constraint symmetric L9 L10.end A1.start
  constraint symmetric L9 L11.start L12.start
  constraint symmetric L9 L11.end A1.end
  constraint symmetric L9 A0 A1
  measures "d20" diameter of A0
  measures "d21" distance of L10 L11
  measures "d22" distance of L3 A0.centre
extrude "Extrude5" cut sketch "Sketch5" against normal through all contours L3 L10 L11 A0 | L5 A1 L12 L13 bodies 1
sketch "Sketch6" plane through (0, 0, 0) normal (-1, 0, 0) x (0, -1, 0)
  line L0 (0, 0) -> (0, 15.9)
  line L1 (0, 15.9) -> (-11.75, 15.9)
  line L2 (-11.75, 15.9) -> (-11.75, 0)
  line L3 (-11.75, 0) -> (0, 0)
  line L4 (-4.075, 5.7) -> (-7.675, 5.7) construction
  line L5 (-7.675, 5.7) -> (-7.675, 4.5) construction
  line L6 (-7.675, 4.5) -> (-4.075, 4.5) construction
  line L7 (-4.075, 4.5) -> (-4.075, 5.7) construction
  line L8 (-5.875, 4.5) -> (-5.875, 0) construction
  circle A0 centre (-5.875, 5.1) radius 0.6
  circle A1 centre (-4.675, 5.1) radius 0.6
  circle A2 centre (-7.075, 5.1) radius 0.6
  dimension "d24" = 1.2
  dimension "d25" = 4.5
  constraint horizontal L4
  constraint vertical L5
  constraint horizontal L6
  constraint vertical L7
  constraint midpoint L6 L8.start
  constraint coincident L3 L8.end
  constraint perpendicular L3 L8
  constraint midpoint L3 L8.end
  constraint tangent L4 A0
  constraint coincident L8.start A0
  constraint tangent L4 A1
  constraint tangent L7 A1
  constraint tangent L6 A1
  constraint tangent L4 A2
  constraint tangent L5 A2
  constraint tangent L6 A2
  constraint tangent A0 A1
  constraint tangent A0 A2
  measures "d24" distance of L4.start L6.end
  measures "d25" distance of L8.start L8.end
extrude "Extrude6" add sketch "Sketch6" along normal blind 7 separate body contours A0 | A2 | A1 makes body 3
equation "d43 = 3.9 mm - 2.2 mm"
named bodies: "Body", "Wires", "Mount"

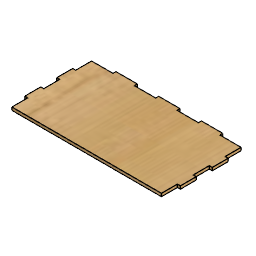
design "Base"
Autodesk Fusion 360 part; units mm, degrees
sketch "Sketch1" plane through (0, 0, 0) normal (0, 0, 1) x (1, 0, 0)
  line L0 (0, 0) -> (150, 0)
  line L1 (150, 0) -> (150, 80)
  line L2 (150, 80) -> (0, 80)
  line L3 (0, 80) -> (0, 0)
  line L4 (150, 64) -> (153, 64)
  line L5 (153, 64) -> (153, 48)
  line L6 (153, 48) -> (150, 48)
  line L7 (150, 32) -> (153, 32)
  line L8 (153, 32) -> (153, 16)
  line L9 (153, 16) -> (150, 16)
  line L10 (153, 32) -> (153, 48) construction
  line L11 (153, 40) -> (150, 40) construction
  line L12 (153, 16) -> (153, 0) construction
  line L13 (153, 0) -> (150, 0) construction
  line L14 (75, 80) -> (75, 0) construction
  line L15 (0, 64) -> (-3, 64)
  line L16 (-3, 64) -> (-3, 48)
  line L17 (-3, 48) -> (0, 48)
  line L18 (0, 32) -> (-3, 32)
  line L19 (-3, 32) -> (-3, 16)
  line L20 (-3, 16) -> (0, 16)
  line L21 (128.5714, 80) -> (128.5714, 83)
  line L22 (128.5714, 83) -> (107.1429, 83)
  line L23 (107.1429, 83) -> (107.1429, 80)
  line L24 (85.7143, 80) -> (85.7143, 83)
  line L25 (85.7143, 83) -> (64.2857, 83)
  line L26 (64.2857, 83) -> (64.2857, 80)
  line L27 (42.8571, 80) -> (42.8571, 83)
  line L28 (42.8571, 83) -> (21.4286, 83)
  line L29 (21.4286, 83) -> (21.4286, 80)
  line L30 (42.8571, 83) -> (64.2857, 83) construction
  line L31 (85.7143, 83) -> (107.1429, 83) construction
  line L32 (128.5714, 83) -> (150, 83) construction
  line L33 (150, 83) -> (150, 80) construction
  line L34 (75, 83) -> (75, 80) construction
  dimension "d9" = 150
  dimension "d10" = 80
  dimension "d40" = 3
  dimension "d44" = 3
  constraint horizontal L0
  constraint vertical L1
  constraint horizontal L2
  constraint vertical L3
  constraint coincident L0.start L3.end
  constraint coincident L1 L4.start
  constraint perpendicular L1 L4
  constraint perpendicular L4 L5
  constraint coincident L1 L6.end
  constraint perpendicular L1 L6
  constraint coincident L1 L7.start
  constraint perpendicular L1 L7
  constraint perpendicular L7 L8
  constraint coincident L1 L9.end
  constraint perpendicular L1 L9
  constraint collinear L5 L8
  constraint equal L5 L10
  constraint equal L8 L10
  constraint midpoint L10 L11.start
  constraint midpoint L1 L11.end
  constraint perpendicular L10 L11
  constraint perpendicular L9 L12
  constraint perpendicular L12 L13
  constraint equal L8 L12
  constraint midpoint L2 L14.start
  constraint midpoint L0 L14.end
  constraint symmetric L4.start L14 L15.start
  constraint symmetric L4.end L14 L15.end
  constraint symmetric L5.end L14 L16.end
  constraint symmetric L6.end L14 L17.end
  constraint symmetric L7.start L14 L18.start
  constraint symmetric L7.end L14 L18.end
  constraint symmetric L8.end L14 L19.end
  constraint symmetric L9.end L14 L20.end
  constraint coincident L2 L21.start
  constraint perpendicular L2 L21
  constraint perpendicular L21 L22
  constraint coincident L2 L23.end
  constraint perpendicular L2 L23
  constraint coincident L2 L24.start
  constraint perpendicular L2 L24
  constraint perpendicular L24 L25
  constraint coincident L2 L26.end
  constraint perpendicular L2 L26
  constraint coincident L2 L27.start
  constraint perpendicular L2 L27
  constraint perpendicular L26 L28
  constraint coincident L2 L29.end
  constraint perpendicular L2 L29
  constraint perpendicular L26 L30
  constraint perpendicular L23 L31
  constraint perpendicular L1 L32
  constraint perpendicular L2 L33
  constraint midpoint L25 L34.start
  constraint equal L22 L32
  constraint equal L22 L31
  constraint equal L25 L31
  constraint equal L25 L30
  constraint equal L28 L30
  constraint perpendicular L2 L34
  measures "d9" distance of L0.start L0.end
  measures "d10" distance of L0.start L2.end
  measures "d40" distance of L8.end L9.end
  measures "d44" distance of L21.start L21.end
extrude "Extrude1" add sketch "Sketch1" along normal blind 3
sketch "Sketch2" plane through (0, 0, 3) normal (0, 0, 1) x (-1, 0, 0)
  line L0 (-150, -64) -> (-150, -80)
  line L1 (-150, -80) -> (-128.5714, -80)
  line L2 (-128.5714, -80) -> (-128.5714, -83)
  line L3 (-128.5714, -83) -> (-107.1429, -83)
  line L4 (-107.1429, -83) -> (-107.1429, -80)
  line L5 (-107.1429, -80) -> (-85.7143, -80)
  line L6 (-85.7143, -80) -> (-85.7143, -83)
  line L7 (-85.7143, -83) -> (-64.2857, -83)
  line L8 (-64.2857, -83) -> (-64.2857, -80)
  line L9 (-64.2857, -80) -> (-42.8571, -80)
  line L10 (-42.8571, -80) -> (-42.8571, -83)
  line L11 (-42.8571, -83) -> (-21.4286, -83)
  line L12 (-21.4286, -83) -> (-21.4286, -80)
  line L13 (-21.4286, -80) -> (0, -80)
  line L14 (0, -80) -> (0, -64)
  line L15 (0, -64) -> (3, -64)
  line L16 (3, -64) -> (3, -48)
  line L17 (3, -48) -> (0, -48)
  line L18 (0, -48) -> (0, -32)
  line L19 (0, -32) -> (3, -32)
  line L20 (3, -32) -> (3, -16)
  line L21 (3, -16) -> (0, -16)
  line L22 (0, -16) -> (0, 0)
  line L23 (0, 0) -> (-150, 0)
  line L24 (-150, 0) -> (-150, -16)
  line L25 (-150, -16) -> (-153, -16)
  line L26 (-153, -16) -> (-153, -32)
  line L27 (-153, -32) -> (-150, -32)
  line L28 (-150, -32) -> (-150, -48)
  line L29 (-150, -48) -> (-153, -48)
  line L30 (-153, -48) -> (-153, -64)
  line L31 (-153, -64) -> (-150, -64)
  line L32 (0, -73) -> (0, -4)
  line L33 (0, -73) -> (-85, -73)
  circle A0 centre (-4.3167, -68.642) radius 1.5875
  circle A1 centre (-4.3196, -8.317) radius 1.5875
  circle A2 centre (-80.6437, -68.6448) radius 1.5875
  circle A3 centre (-23.876, -42.417) radius 1.651
  dimension "d1" = 69
  dimension "d2" = 85
  dimension "d3" = 3.175
  dimension "d4" = 6.134
  dimension "d5" = 3.175
  dimension "d6" = 6.107
  dimension "d7" = 3.175
  dimension "d8" = 6.16
  dimension "d13" = 76.327
  dimension "d14" = 60.325
  dimension "d15" = 3.302
  dimension "d16" = 30.583
  dimension "d17" = 23.876
  dimension "d18" = 34.1
  dimension "d19" = 26.2278
  dimension "d29" = 12
  dimension "d17" = 23.876
  constraint coincident L14 L32.start
  constraint perpendicular L15 L32
  constraint perpendicular L32 L33
  measures "d1" distance of L32.start L32.end
  measures "d2" distance of L32.start L33.end
  measures "d3" diameter of A0
  measures "d4" distance of L32.start A0.centre
  measures "d5" diameter of A1
  measures "d6" distance of L32.end A1.centre
  measures "d7" diameter of A2
  measures "d13" horizontal distance of A0.centre A2.centre
  measures "d14" vertical distance of A0.centre A1.centre
  measures "d15" diameter of A3
  measures "d16" vertical distance of L32.start A3.centre
  measures "d17" distance of L32 A3.centre
  measures "d18" vertical distance of A1.centre A3.centre
  measures "d19" vertical distance of A2.centre A3.centre
  measures "d29" distance of L21 L32.end

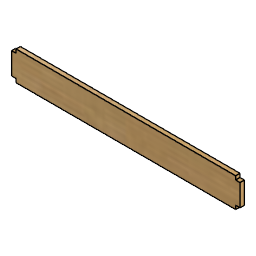
design "Front Brace"
Autodesk Fusion 360 part; units mm, degrees
sketch "Sketch4" plane through (0, 3, 0) normal (0, -1, 0) x (1, 0, 0)
  line L0 (0, 130) -> (0, 145)
  line L1 (0, 145) -> (-3, 145)
  line L2 (-3, 145) -> (-3, 130)
  line L3 (-3, 130) -> (0, 130)
  line L4 (150, 145) -> (150, 130)
  line L5 (150, 130) -> (153, 130)
  line L6 (153, 130) -> (153, 145)
  line L7 (153, 145) -> (150, 145)
  line L8 (0, 145) -> (0, 147.5)
  line L9 (0, 147.5) -> (150, 147.5)
  line L10 (150, 147.5) -> (150, 145)
  line L11 (150, 130) -> (150, 127.5)
  line L12 (150, 127.5) -> (0, 127.5)
  line L13 (0, 127.5) -> (0, 130)
  dimension "d59" = 20
  constraint coincident L0.end L1.start
  constraint perpendicular L1 L8
  constraint perpendicular L4 L9
  constraint coincident L4.start L7.end
  constraint perpendicular L7 L10
  constraint coincident L4.end L5.start
  constraint perpendicular L5 L11
  constraint perpendicular L0 L12
  constraint coincident L0.start L3.end
  constraint perpendicular L3 L13
  constraint equal L8 L13
  measures "d59" distance of L9 L12
extrude "Extrude2" add sketch "Sketch4" along normal blind 3

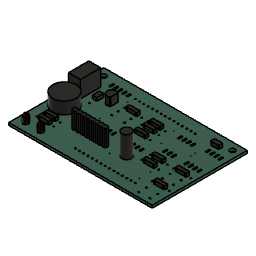
design "IO Daughter Board"
Autodesk Fusion 360 part; units mm, degrees
sketch "Outline" plane through (0, 0, 0) normal (0, 0, 1) x (1, 0, 0)
  line L0 (0, 0) -> (0, 56.3)
  arc A0 (0, 56.3381) -> (0, 56.2619) centre (0, 56.3) ccw
  line L1 (85, 56.3) -> (85, 0)
  arc A1 (85.0381, 56.3) -> (84.9619, 56.3) centre (85, 56.3) ccw
  arc A2 (0.0381, 56.3) -> (-0.0381, 56.3) centre (0, 56.3) ccw
  arc A3 (-0.0381, 0) -> (0.0381, 0) centre (0, 0) ccw
  line L2 (0, 56.3) -> (85, 56.3)
  arc A4 (0, 0.0381) -> (0, -0.0381) centre (0, 0) ccw
  arc A5 (85, 56.2619) -> (85, 56.3381) centre (85, 56.3) ccw
  arc A6 (85, -0.0381) -> (85, 0.0381) centre (85, 0) ccw
  line L3 (85, 0) -> (0, 0)
  arc A7 (84.9619, 0) -> (85.0381, 0) centre (85, 0) ccw